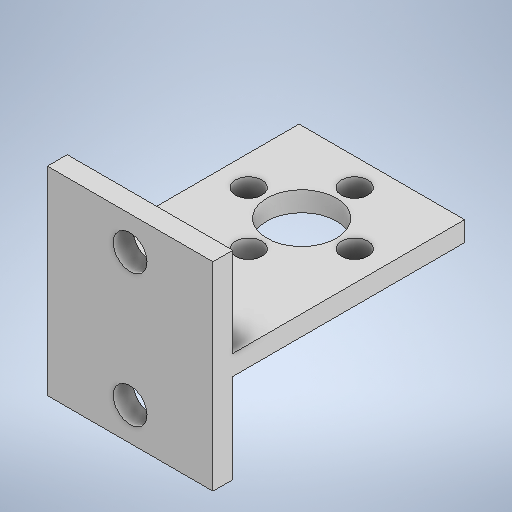
# Autodesk Inventor part: LeadCarriageConnector
Saved by Autodesk Inventor 2025.2 (Build 292293000, 293)
## iProperties
Created: 2025-07-19
Part Number: LeadCarriageConnector
Material: Generic
Document SubType Name: Modeling
Designer: Simon
Density: 1 g/cm^3
Appearance: Default
Author: Simon
Autodesk Inventor part; units mm, degrees
ref_plane "YZ Plane" through (0, 0, 0) normal (1, 0, 0) x (0, 1, 0)
ref_plane "XZ Plane" through (0, 0, 0) normal (0, 1, 0) x (-1, 0, 0)
ref_plane "XY Plane" through (0, 0, 0) normal (0, 0, 1) x (1, 0, 0)
sketch "Sketch1" plane through (0, 0, 0) normal (0, 0, 1) x (1, 0, 0)
  line L0 (12.5, 15) -> (-12.5, 15)
  line L1 (-12.5, 15) -> (-12.5, -15)
  line L2 (-12.5, -15) -> (12.5, -15)
  line L3 (12.5, -15) -> (12.5, 15)
  line L4 (12.5, 15) -> (-12.5, -15) construction
  line L5 (-12.5, 15) -> (12.5, -15) construction
  point P0 (0, 0)
  dimension "d0" = 25
  dimension "d1" = 30
  constraints: 12 end point, 2 midpoint, 2 parallel, 1 horizontal, 1 perpendicular
  measures "d0" distance of L2.end L1.end
  measures "d1" distance of L1.end L0.end
extrude "Extrusion1" add sketch "Sketch1" against normal blind 3
sketch "Sketch2" plane through (0, 0, -3) normal (0, 0, -1) x (-1, 0, 0)
  line L0 (12.5, -15) -> (12.5, 15) projected
  line L1 (-12.5, 1.5) -> (12.5, 1.5)
  line L2 (12.5, 1.5) -> (12.5, -1.5)
  line L3 (12.5, -1.5) -> (-12.5, -1.5)
  line L4 (-12.5, -1.5) -> (-12.5, 1.5)
  line L5 (-12.5, 1.5) -> (12.5, -1.5) construction
  line L6 (12.5, 1.5) -> (-12.5, -1.5) construction
  point P0 (0, 0)
  dimension "d4" = 3
  constraints: 12 end point, 2 midpoint, 2 parallel, 1 horizontal, 1 perpendicular, 1 point on line
  measures "d4" distance of L1.end L2.end
extrude "Extrusion2" add sketch "Sketch2" along normal blind 35
sketch "Sketch3" plane through (0, 0, 0) normal (0, 0, 1) x (1, 0, 0)
  line L0 (0, 10) -> (0, -10)
  circle A0 centre (0, 10) radius 2.55
  circle A1 centre (0, -10) radius 2.55
  point P0 (0, 0)
  dimension "d7" = 20
  dimension "d8" = 5.1
  dimension "d9" = 5.1
  constraints: 2 centre point, 2 coincident, 2 end point, 1 midpoint, 1 vertical
  measures "d7" distance of L0.start L0.end
  measures "d8" diameter of A0
  measures "d9" diameter of A1
extrude "Extrusion3" cut sketch "Sketch3" against normal through all
sketch "Sketch4" plane through (-12.5, 1.5, -3) normal (0, 1, 0) x (1, 0, 0)
  line L0 (9.95, 0) -> (15.05, 0) projected
  line L1 (12.5, 0) -> (12.5, 22.896)
  circle A0 centre (12.5, 22.896) radius 5.25
  circle A1 centre (12.5, 22.896) radius 8
  circle A2 centre (12.5, 14.896) radius 2
  circle A3 centre (20.5, 22.896) radius 2
  circle A4 centre (12.5, 30.896) radius 2
  circle A5 centre (4.5, 22.896) radius 2
  point P0 (12.5, -3)
  dimension "d14" = 16
  dimension "d12" = 22.896
  dimension "d13" = 10.5
  dimension "d15" = 4
  dimension "d18" = 360
  constraints: 5 centre point, 2 coincident, 2 end point, 1 midpoint, 1 point on line, 1 vertical, 1 vertical alignment, 11 other
  measures "d12" distance of L1.start L1.end
  measures "d13" diameter of A0
  measures "d15" diameter of A2
extrude "Extrusion4" cut sketch "Sketch4" against normal through all contours A2 A1 L1 | L1 A1 A2 | A1 A2 L1 | L1 A2 A1 | A0 | A5 A1 | A1 A5 | A3 A1 | A1 A3 | A4 A1 | A1 A4
body "Solid1"
